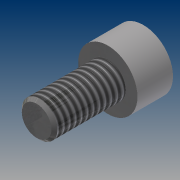
# Autodesk Inventor part: M6_12mm
Saved by Autodesk Inventor 2015 (Build 190159000, 159)
## iProperties
Created: 2015-03-27
Part Number: M6_12mm
Material: Steel, Carbon
Document SubType Name: Modeling
Designer: nfitch
Density: 7.85 g/cm^3
Appearance: Semi-Polished
Mass: 5.07153 g
Surface Area: 6.60754 cm^2
Volume: 0.646055 cm^3
Author: nfitch
Autodesk Inventor part; units mm, degrees
ref_plane "YZ Plane" through (0, 0, 0) normal (1, 0, 0) x (0, 1, 0)
ref_plane "XZ Plane" through (0, 0, 0) normal (0, 1, 0) x (-1, 0, 0)
ref_plane "XY Plane" through (0, 0, 0) normal (0, 0, 1) x (1, 0, 0)
sketch "Sketch1" plane through (0, 0, 0) normal (0, 1, 0) x (-1, 0, 0)
  circle A0 centre (0, 0) radius 3
  dimension "d0" = 6
  constraints: 1 centre point, 1 coincident
  measures "d0" diameter of A0
extrude "Extrusion1" add sketch "Sketch1" along normal blind 12
thread "Thread1" size "M6x1" class "6g" standard "ANSI Metric M Profile" full length
chamfer "Chamfer1" distance 0.5 angle 45 1 edges at (3, 0, 0)
sketch "Sketch2" plane through (0, 12, 0) normal (0, 1, 0) x (1, 0, 0)
  circle A0 centre (0, 0) radius 5
  dimension "d8" = 10
  constraints: 1 centre point, 1 coincident
  measures "d8" diameter of A0
extrude "Extrusion2" add sketch "Sketch2" along normal blind 6
sketch "Sketch3" plane through (0, 18, 0) normal (0, 1, 0) x (1, 0, 0)
  line L0 (-3.4231, 1.9737) -> (-0.0023, 3.9513)
  line L1 (-0.0023, 3.9513) -> (3.4208, 1.9776)
  line L2 (3.4208, 1.9776) -> (3.4231, -1.9737)
  line L3 (3.4231, -1.9737) -> (0.0023, -3.9513)
  line L4 (0.0023, -3.9513) -> (-3.4208, -1.9776)
  line L5 (-3.4208, -1.9776) -> (-3.4231, 1.9737)
  point P0 (0, 0)
  point P1 (0, 0)
  constraints: 12 end point, 1 coincident, 13 other
extrude "Extrusion3" cut sketch "Sketch3" against normal blind 4
body "Solid1"
